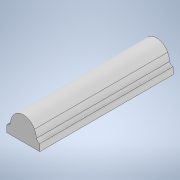
# Autodesk Inventor part: gt2-2
Saved by Autodesk Inventor 2020 (Build 240168000, 168)
## iProperties
Created: 2021-02-20
Part Number: gt2-2
Material: Generic
Document SubType Name: Modeling
Designer: AOB
Mass: 0.00716311 g
Surface Area: 0.289558 cm^2
Volume: 0.00716311 cm^3
Density: 1 g/cm^3
Appearance: Default
Author: AOB
Autodesk Inventor part; units mm, degrees
ref_plane "YZ Plane" through (0, 0, 0) normal (1, 0, 0) x (0, 1, 0)
ref_plane "XZ Plane" through (0, 0, 0) normal (0, 1, 0) x (-1, 0, 0)
ref_plane "XY Plane" through (0, 0, 0) normal (0, 0, 1) x (1, 0, 0)
sketch "Sketch1" plane through (-205.541, 0, 0) normal (0, 0, 1) x (1, 0, 0)
  arc A0 (62.3925, -4.576) -> (62.6535, -4.3678) centre (62.4202, -4.343) ccw
  line L0 (62.3925, -4.576) -> (62.1418, -4.5462)
  line L1 (62.3925, -4.534) -> (62.3925, -4.576)
  line L2 (65.7271, -4.551) -> (65.7271, -4.576)
  arc A1 (1.4989, -4.1378) -> (0.5011, -4.1378) centre (1, -4.381) ccw
  arc A2 (0.5011, -4.1378) -> (0.4085, -4.4456) centre (1.4, -4.576) ccw
  arc A3 (0.2598, -4.576) -> (0.4085, -4.4456) centre (0.2598, -4.426) ccw
  arc A4 (1.5915, -4.4456) -> (1.4989, -4.1378) centre (0.6, -4.576) ccw
  arc A5 (1.5915, -4.4456) -> (1.7402, -4.576) centre (1.7402, -4.426) ccw
  line L3 (0.2598, -4.891) -> (0.2598, -4.576)
  line L4 (1.7402, -4.576) -> (1.7402, -4.891)
  line L5 (0.2598, -4.891) -> (1.7402, -4.891)
  point P0 (-0.2846, 5.3732)
  dimension "d12" = 0.555
  dimension "d13" = 1
  dimension "d14" = 1
  dimension "d15" = 0.15
  dimension "d16" = 0.15
  dimension "d18" = 0.195
  constraints: 12 end point, 12 point on circle, 6 centre point
  measures "d12" radius of A1
  measures "d13" radius of A2
  measures "d14" radius of A4
  measures "d15" radius of A3
  measures "d16" radius of A5
  measures "d18" vertical distance of L4.start A1.centre
extrude "Extrusion1" add sketch "Sketch1" along normal blind 6
body "Solid1"
